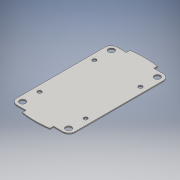
# Autodesk Inventor part: board_outline
Saved by Autodesk Inventor 2016 (Build 200138000, 138)
## iProperties
Created: 2019-09-21
Part Number: board_outline
Material: Типовые
Document SubType Name: Modeling
Designer: Nurekengoi
Density: 1 g/cm^3
Appearance: По умолчанию
Author: Nurekengoi
Autodesk Inventor part; units mm, degrees
ref_plane "YZ Plane" through (0, 0, 0) normal (1, 0, 0) x (0, 1, 0)
ref_plane "XZ Plane" through (0, 0, 0) normal (0, 1, 0) x (-1, 0, 0)
ref_plane "XY Plane" through (0, 0, 0) normal (0, 0, 1) x (1, 0, 0)
sketch "Эскиз3" plane through (0, 0, 0) normal (0, 0, 1) x (1, 0, 0)
  circle A0 centre (-21, 40.5) radius 2.7
  line L0 (0, 0) -> (8.3957, 0)
  line L1 (0, 0) -> (0, -7.8184)
  circle A1 centre (21, 40.5) radius 2.7
  circle A2 centre (-21, -40.5) radius 2.7
  circle A3 centre (21, -40.5) radius 2.7
  circle A4 centre (-21, 25) radius 1.75
  circle A5 centre (21, 25) radius 1.75
  circle A6 centre (-21, -25) radius 1.75
  circle A7 centre (21, -25) radius 1.75
  line L2 (-26.5, 40.332) -> (-26.5, 0)
  arc A8 (-21.3, 45.6934) -> (-26.5, 40.332) centre (-21, 40.2) ccw
  line L3 (-21.3, 45.6934) -> (-12.5, 45.6934)
  line L4 (-12.5, 45.6934) -> (-12.5, 48.9877)
  arc A9 (0, 49.934) -> (-12.5, 48.9877) centre (0, -33.098) ccw
  line L5 (-26.5, -40.332) -> (-26.5, 0)
  arc A10 (-26.5, -40.332) -> (-21.3, -45.6934) centre (-21, -40.2) ccw
  line L6 (-21.3, -45.6934) -> (-12.5, -45.6934)
  line L7 (-12.5, -45.6934) -> (-12.5, -48.9877)
  arc A11 (-12.5, -48.9877) -> (0, -49.934) centre (0, 33.098) ccw
  line L8 (26.5, 40.332) -> (26.5, 0)
  arc A12 (26.5, 40.332) -> (21.3, 45.6934) centre (21, 40.2) ccw
  line L9 (21.3, 45.6934) -> (12.5, 45.6934)
  line L10 (12.5, 45.6934) -> (12.5, 48.9877)
  arc A13 (12.5, 48.9877) -> (0, 49.934) centre (0, -33.098) ccw
  line L11 (26.5, -40.332) -> (26.5, 0)
  arc A14 (21.3, -45.6934) -> (26.5, -40.332) centre (21, -40.2) ccw
  line L12 (21.3, -45.6934) -> (12.5, -45.6934)
  arc A15 (0, -49.934) -> (12.5, -48.9877) centre (0, 33.098) ccw
  line L13 (12.5, -45.6934) -> (12.5, -48.9877)
  circle A16 centre (-10, 38.5) radius 1.75
  circle A17 centre (10, 38.5) radius 1.75
  circle A18 centre (-10, -38.5) radius 1.75
  circle A19 centre (10, -38.5) radius 1.75
  dimension "d19" = 5.4
  dimension "d20" = 42
  dimension "d21" = 81
  dimension "d22" = 3.5
  dimension "d23" = 42
  dimension "d24" = 50
  dimension "d25" = 0
  dimension "d26" = 53
  dimension "d27" = 0.168
  dimension "d28" = 0
  dimension "d29" = 0.3
  dimension "d31" = 12.5
  dimension "d32" = 73.298
  dimension "d33" = 83.032
  dimension "d34" = 0
  dimension "d35" = 0.3
  dimension "d38" = 3.5
  dimension "d39" = 20
  dimension "d40" = 77
  constraints: 28 end point, 20 centre point, 16 point on circle, 14 symmetric about line, 7 other
  measures "d19" diameter of A0
  measures "d20" diameter of A0.centre L1
  measures "d21" diameter of A0.centre L0
  measures "d22" diameter of A4
  measures "d23" diameter of A4.centre L1
  measures "d24" diameter of A4.centre L0
  measures "d25" vertical distance of L0.start L2.end
  measures "d26" diameter of L2 L1
  measures "d27" vertical distance of L2.start A0.centre
  measures "d28" horizontal distance of A0.centre A8.centre
  measures "d29" distance of A0.centre A8.centre
  measures "d31" distance from line of L0.start L4
  measures "d32" vertical distance of A8.centre A9.centre
  measures "d33" radius of A9
  measures "d34" horizontal distance of L0.start A9.centre
  measures "d35" horizontal distance of L3.start A0.centre
  measures "d38" diameter of A16
  measures "d39" diameter of A16.centre L1
  measures "d40" diameter of A16.centre L0
extrude "Тело" add sketch "Эскиз3" along normal blind 1 contours A8 L3 L4 A9 A13 L10 L9 A12 L8 L11 A14 L12 L13 A15 A11 L7 L6 A10 L5 L2 | A16 | A17 | A18 | A19
